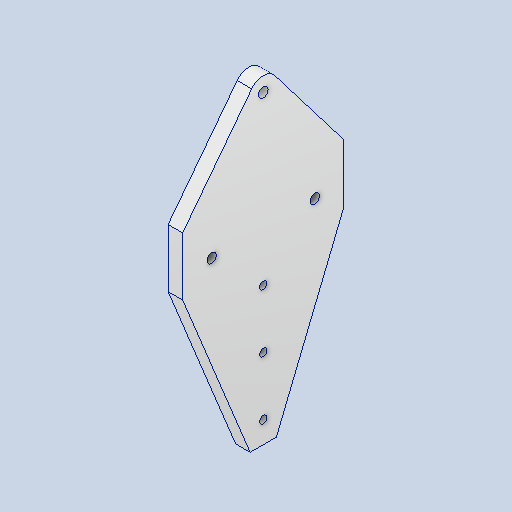
# Autodesk Inventor part: odom_v1_Plate_1
Saved by Autodesk Inventor 2025.2 (Build 292293000, 293)
## iProperties
Created: 2025-03-30
Part Number: odom_v1_Plate_1
Material: アルミニウム 6061
Document SubType Name: Modeling
Designer: haruy
Density: 2.7 g/cm^3
Appearance: アルミニウム - フラット
Author: haruy
Autodesk Inventor part; units mm, degrees
ref_plane "YZ Plane" through (0, 0, 0) normal (1, 0, 0) x (0, 1, 0)
ref_plane "XZ Plane" through (0, 0, 0) normal (0, 1, 0) x (-1, 0, 0)
ref_plane "XY Plane" through (0, 0, 0) normal (0, 0, 1) x (1, 0, 0)
derived "odom_v1_Sketch_Base.ipt"
sketch "スケッチ1" plane through (300, 0, 0) normal (1, 0, 0) x (0, 1, 0)
  line L0 (0, 0) -> (20, 0)
  line L1 (20, 0) -> (20, -192.6893)
  line L2 (20, -192.6893) -> (0, -192.6893)
  line L3 (0, -192.6893) -> (0, 0) construction
  line L4 (-77, 0) -> (-77, -265.1297)
  circle A0 centre (7.5, -57.9764) radius 1.6
  circle A1 centre (7.5, -93.4764) radius 1.6
  line L5 (-20, -52.2264) -> (-66, -52.2264)
  line L6 (-66, -52.2264) -> (-66, -57.2264)
  line L7 (-66, -57.2264) -> (-20, -57.2264) construction
  line L8 (-20, -57.2264) -> (-20, -52.2264)
  line L9 (-20, -94.2264) -> (-66, -94.2264) construction
  line L10 (-66, -94.2264) -> (-66, -99.2264)
  line L11 (-66, -99.2264) -> (-20, -99.2264) construction
  line L12 (-20, -99.2264) -> (-20, -94.2264) construction
  line L13 (-19.371, -66.7264) -> (-77, -66.7264)
  line L14 (-77, -66.7264) -> (-77, -84.7264)
  line L15 (-77, -84.7264) -> (-19.371, -84.7264)
  line L16 (-19.371, -84.7264) -> (-19.371, -66.7264)
  line L17 (-41.1855, -57.2264) -> (-55.1855, -57.2264)
  line L18 (-55.1855, -57.2264) -> (-55.1855, -58.0264)
  line L19 (-55.1855, -58.0264) -> (-41.1855, -58.0264)
  line L20 (-41.1855, -58.0264) -> (-41.1855, -57.2264)
  line L21 (-48.1855, -66.7264) -> (-48.1855, -84.7264)
  line L22 (-55.1855, -94.2264) -> (-41.1855, -94.2264)
  line L23 (-41.1855, -94.2264) -> (-41.1855, -93.4264)
  line L24 (-41.1855, -93.4264) -> (-55.1855, -93.4264)
  line L25 (-55.1855, -93.4264) -> (-55.1855, -94.2264)
  circle A2 centre (48, -75.7264) radius 1.65
  circle A3 centre (-17, -75.7264) radius 2
  line L26 (48, -75.7264) -> (-17, -75.7264) construction
  line L27 (33.5, -67.2264) -> (-12, -67.2264) construction
  line L28 (-12, -67.2264) -> (-12, -84.2264)
  line L29 (-12, -84.2264) -> (33.5, -84.2264)
  line L30 (33.5, -84.2264) -> (33.5, -67.2264) construction
  line L31 (-12, -73.7264) -> (-20, -73.7264)
  line L32 (-20, -73.7264) -> (-20, -77.7264)
  line L33 (-20, -77.7264) -> (-12, -77.7264)
  line L34 (-12, -77.7264) -> (-12, -73.7264)
  line L35 (-2, -71.2264) -> (-57, -71.2264)
  line L36 (-57, -71.2264) -> (-57, -80.2264)
  line L37 (-57, -80.2264) -> (-2, -80.2264)
  line L38 (-2, -80.2264) -> (-2, -71.2264)
  circle A4 centre (-9.5, -75.7264) radius 1.25
  circle A5 centre (-29.5, -75.7264) radius 1.25
  circle A6 centre (-49.5, -75.7264) radius 1.25
  line L39 (-52, -65.7264) -> (-22, -65.7264)
  line L40 (-22, -65.7264) -> (-22, -85.7264)
  line L41 (-22, -85.7264) -> (-52, -85.7264)
  line L42 (-52, -85.7264) -> (-52, -65.7264)
  line L43 (20, -47.9764) -> (0, -47.9764)
  line L44 (0, -47.9764) -> (-57, -71.2264)
  circle A7 centre (48, -75.7264) radius 5
  line L45 (20, -103.4764) -> (0, -103.4764) construction
  line L46 (53, -75.7264) -> (53, -103.4764) construction
  line L47 (0, -103.4764) -> (-14.7581, -103.4764) construction
  line L48 (-57, -80.2264) -> (47.9762, -80.7264)
  line L49 (-43, -52.2264) -> (-43, -57.2264)
  circle A8 centre (-33, -54.7264) radius 1.25
  line L50 (-29.5, -75.7264) -> (-49.5, -75.7264)
  circle A9 centre (-53, -54.7264) radius 1.25
  circle A10 centre (-53, -96.7264) radius 1.25
  circle A11 centre (-33, -96.7264) radius 1.25
  line L51 (48, -70.7264) -> (20, -70.7264)
  line L52 (20, -47.9764) -> (51.0408, -71.7573)
  line L53 (20, -103.4764) -> (51.0408, -79.6955)
  line L54 (20, -103.4764) -> (0, -103.4764)
  line L55 (-2, -71.2264) -> (0, -71.2264)
  line L56 (-2, -80.2264) -> (0, -80.2264)
  line L57 (0, -103.4764) -> (-57, -80.2264)
  point P0 (44.0583, -72.6502)
  point P1 (20, -80.5931)
  point P2 (-48.1855, -80.2264)
  point P3 (-48.1855, -80.2684)
  point P4 (-52, -80.2502)
  point P5 (-52, -80.2264)
  dimension "d1" = 10
  dimension "d2" = 10
  dimension "d3" = 10
  measures "d1" distance from line of L43 A0.centre
  measures "d2" diameter of A7
  measures "d3" distance from line of A1.centre L45
extrude "押し出し1" add sketch "スケッチ1" against normal blind 5 contours L52 A7 L51 L1 | L1 L48 L28 L37 L38 L35 L16 L13 L40 L39 L44 L43 | L51 A7 L48 L1 | A7 | L48 A7 L53 L1 | L1 L29 L28 L48 | L1 L54 L57 L41 L40 L15 L16 L48 L28 L29 | L48 L16 L37 L28 | L39 L40 L13 L44 | L37 L16 L33 L28 | L28 L35 L38 L37 | L48 L40 L37 L16 | L16 L15 L40 L48 | L13 L40 L35 L21 L44 | L33 A3 L31 L28 | L37 L40 L35 L16 L31 L32 L33 | L48 L21 L37 L40 | L40 L15 L57 L21 L48 | L13 L16 L35 L40 | L21 L35 L42 L44 | L57 L15 L40 L41 | L31 L16 L35 L28 | L33 L16 L31 A3 | A3 | L33 L32 L31 L16 | L37 L21 L35 L40 | L48 L42 L37 L21 | L21 L57 L42 L48 | L42 L35 L44 | L21 L37 L42 L35 | L48 L37 L42 | L42 L57 L48 | L42 L37 L36 L35
